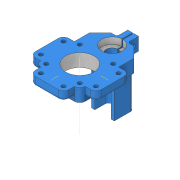
# Autodesk Inventor part: 1 gear box base
Saved by Autodesk Inventor 2020 (Build 240168000, 168)
## iProperties
Created: 2018-08-14
Part Number: 1 gear box base
Material: Generic
Document SubType Name: Modeling
Designer: mrbeh
Density: 1 g/cm^3
Appearance: Default
Author: mrbeh
Autodesk Inventor part; units mm, degrees
ref_plane "YZ Plane" through (0, 0, 0) normal (1, 0, 0) x (0, 1, 0)
ref_plane "XZ Plane" through (0, 0, 0) normal (0, 1, 0) x (-1, 0, 0)
ref_plane "XY Plane" through (0, 0, 0) normal (0, 0, 1) x (1, 0, 0)
sketch "Sketch1" plane through (0, 0, 0) normal (0, 1, 0) x (-1, 0, 0)
  line L0 (0, 0) -> (42, 0)
  line L1 (42, 0) -> (42, -60)
  line L2 (42, -60) -> (0, -60)
  line L3 (0, -60) -> (0, 0)
  dimension "d0" = 42
  dimension "d1" = 60
  constraints: 8 end point, 2 parallel, 1 horizontal, 1 perpendicular
  measures "d0" distance of L1.end L2.end
  measures "d1" distance of L0.end L1.end
extrude "Extrusion1" add sketch "Sketch1" along normal blind 12
sketch "Sketch2" plane through (0, 12, 0) normal (0, 1, 0) x (1, 0, 0)
  circle A0 centre (-5, 5) radius 1.8
  point P0 (0, 0)
  dimension "d4" = 3.6
  constraints: 1 centre point
  measures "d4" diameter of A0
extrude "Extrusion2" cut sketch "Sketch2" against normal blind 12
pattern_linear "Rectangular Pattern1" count 2 spacing 31 along (0, 0, -1) count 2 spacing 31 along (-1, 0, 0) of "Extrusion2"
sketch "Sketch3" plane through (0, 12, 0) normal (0, 1, 0) x (1, 0, 0)
  circle A0 centre (-20.5, 20.5) radius 11.5
  point P0 (0, 0)
  dimension "d13" = 23
  constraints: 1 centre point
  measures "d13" diameter of A0
extrude "Extrusion3" cut sketch "Sketch3" against normal blind 12
sketch "Sketch5" plane through (0, 0, 0) normal (0, -1, 0) x (1, 0, 0)
  line L0 (-42, -60) -> (0, -60) projected
  line L1 (0, -31.65) -> (-42, -31.65)
  line L2 (-42, -31.65) -> (-42, -60)
  line L3 (-42, -60) -> (0, -60)
  line L4 (0, -60) -> (0, -31.65)
  point P0 (0, 0)
  constraints: 8 end point, 2 parallel, 1 horizontal, 1 perpendicular
extrude "Extrusion5" add sketch "Sketch5" along normal blind 39.25
sketch "Sketch6" plane through (0, 12, 0) normal (0, 1, 0) x (1, 0, 0)
  line L0 (-25.5, 60) -> (-25.5, 70)
  line L1 (-25.5, 70) -> (-15.5, 70)
  line L2 (-15.5, 70) -> (-15.5, 60)
  line L3 (-42, 60) -> (0, 60) projected
  line L4 (-25.5, 60) -> (-15.5, 60)
  point P0 (0, 0)
  dimension "d21" = 10
  dimension "d23" = 10
  constraints: 8 end point, 2 point on line, 1 parallel
  measures "d21" distance of L0.end L1.end
  measures "d23" distance of L1.end L2.end
extrude "Extrusion6" add sketch "Sketch6" against normal blind 12
sketch "Sketch7" plane through (0, 12, 0) normal (0, 1, 0) x (1, 0, 0)
  line L0 (-20, 60.5) -> (-21, 60.5)
  line L1 (-21, 60.5) -> (-21, 81.6021)
  line L2 (-21, 81.6021) -> (-20, 81.6021)
  line L3 (-20, 81.6021) -> (-20, 60.5)
  point P0 (0, 0)
  dimension "d26" = 1
  constraints: 8 end point, 2 parallel, 1 horizontal, 1 perpendicular
  measures "d26" distance of L1.end L2.end
extrude "Extrusion7" cut sketch "Sketch7" against normal blind 12
sketch "Sketch10" plane through (-25.5, 12, -70) normal (-1, 0, 0) x (0, 0, 1)
  circle A0 centre (5, -6) radius 1.8
  point P0 (70, -12)
  dimension "d35" = 3.6
  constraints: 1 centre point
  measures "d35" diameter of A0
extrude "Extrusion10" cut sketch "Sketch10" against normal blind 10
sketch "Sketch12" plane through (0, 12, 0) normal (0, 1, 0) x (1, 0, 0)
  line L0 (-42, 60) -> (-42, 0) projected
  line L1 (-42, 60) -> (0, 60) projected
  line L2 (-42, 0) -> (-41, 0)
  line L3 (-41, 0) -> (-41, 60)
  line L4 (-41, 60) -> (-42, 60)
  line L5 (-42, 60) -> (-42, 0)
  point P0 (0, 0)
  dimension "d44" = 1
  constraints: 8 end point, 2 parallel, 1 horizontal, 1 perpendicular, 1 point on line
  measures "d44" distance of L4.end L3.end
extrude "Extrusion12" cut sketch "Sketch12" against normal blind 70
fillet "Fillet1" radius 2 2 edges at (-15.5, 6, -60) (-25.5, 6, -60)
fillet "Fillet3" radius 5 2 edges at (0, 6, 0) (-41, 6, 0)
chamfer "Chamfer1" distance 10 angle 45 2 edges at (0, -13.625, -60) (-41, -13.625, -60)
sketch "Sketch14" plane through (0, -39.25, -31.65) normal (0, 0, 1) x (1, 0, 0)
  line L0 (0, 39.25) -> (-5, 39.25) projected
  line L1 (0, 39.25) -> (-10, 39.25)
  line L2 (-10, 39.25) -> (-10, 3.175)
  line L3 (0, 3.175) -> (0, 39.25)
  line L4 (0, 39.25) -> (0, 0) projected
  line L5 (-10, 39.25) -> (0, 39.25)
  line L6 (0, 39.25) -> (0, 0)
  line L7 (0, 0) -> (-10, 0)
  line L8 (-10, 0) -> (-10, 39.25)
  dimension "d57" = 10
  constraints: 14 end point, 3 parallel, 2 horizontal, 2 perpendicular
  measures "d57" distance of L3.start L2.end
extrude "Extrusion14" cut sketch "Sketch14" against normal blind 30
ref_plane "Work Plane1" through (-20.5, 0, -5) normal (1, 0, 0) x (0, 0, -1)
mirror "Mirror1" about plane through (-20.5, 0, -5) normal (1, 0, 0) of "Extrusion14"
sketch "Sketch15" plane through (0, -39.25, 0) normal (0, -1, 0) x (1, 0, 0)
  line L0 (-31, -31.65) -> (-23.3156, -31.65) projected
  line L1 (-13, -31.65) -> (-28, -31.65)
  line L2 (-28, -31.65) -> (-28, -54.65)
  line L3 (-28, -54.65) -> (-13, -54.65)
  line L4 (-13, -54.65) -> (-13, -31.65)
  point P0 (0, 0)
  point P1 (-31, -41.65)
  point P2 (-10, -41.65)
  dimension "d61" = 15
  dimension "d62" = 23
  constraints: 8 end point, 2 parallel, 1 horizontal, 1 perpendicular, 2 other
  measures "d61" distance of L3.end L2.end
  measures "d62" distance of L2.end L1.end
extrude "Extrusion15" cut sketch "Sketch15" against normal blind 36
fillet "Fillet5" radius 3 4 edges at (-10, -19.625, -60) (-28, -21.25, -54.65) (-13, -21.25, -54.65) (-31, -19.625, -60)
sketch "Sketch16" plane through (0, 0, 0) normal (0, -1, 0) x (1, 0, 0)
  line L0 (-41, -50) -> (-41, -5) projected
  line L1 (0, 0) -> (-41, 0)
  line L2 (-41, 0) -> (-41, -42)
  line L3 (-41, -42) -> (0, -42)
  line L4 (0, -42) -> (0, 0)
  dimension "d66" = 42
  constraints: 8 end point, 2 parallel, 1 horizontal, 1 perpendicular, 1 point on line
  measures "d66" distance of L2.end L1.end
extrude "Extrusion16" cut sketch "Sketch16" along normal blind 50
sketch "Sketch17" plane through (0, 12, 0) normal (0, 1, 0) x (1, 0, 0)
  circle A0 centre (-20.5, 50.5) radius 8.55
  point P0 (0, 0)
  dimension "d69" = 17.1
  constraints: 1 centre point
  measures "d69" diameter of A0
extrude "Extrusion17" cut sketch "Sketch17" against normal blind 12.5
sketch "Sketch18" plane through (0, 12, 0) normal (0, 1, 0) x (1, 0, 0)
  line L0 (-25.5, 70) -> (-21, 70) projected
  line L1 (-21, 70) -> (-20, 70)
  line L2 (-20, 70) -> (-20, 46.0375)
  line L3 (-20, 46.0375) -> (-21, 46.0375)
  line L4 (-21, 46.0375) -> (-21, 70)
  point P0 (0, 0)
  constraints: 8 end point, 2 parallel, 1 horizontal, 1 perpendicular
extrude "Extrusion18" cut sketch "Sketch18" against normal blind 12.5
sketch "Sketch20" plane through (0, 12, 0) normal (0, 1, 0) x (1, 0, 0)
  line L0 (0, 50) -> (0, 5) projected
  line L1 (0, 36) -> (10, 36)
  line L2 (10, 36) -> (10, 5)
  line L3 (10, 5) -> (0, 5)
  line L4 (0, 5) -> (0, 36)
  point P0 (0, 0)
  dimension "d76" = 10
  constraints: 8 end point, 2 parallel, 1 horizontal, 1 perpendicular, 1 point on line
  measures "d76" distance of L2.end L3.end
extrude "Extrusion19" add sketch "Sketch20" against normal blind 8
pattern_circular "Circular Pattern2" count 3 over 180 about axis through (-20.5, 12, -20.5) along (0, -1, 0) of "Extrusion19"
sketch "Sketch21" plane through (0, 12, 0) normal (0, 1, 0) x (1, 0, 0)
  circle A0 centre (5, 31) radius 1.8
  point P0 (0, 0)
  dimension "d82" = 3.6
  constraints: 1 centre point
  measures "d82" diameter of A0
extrude "Extrusion20" cut sketch "Sketch21" against normal blind 8
pattern_linear "Rectangular Pattern2" count 2 spacing 21 along (0, 0, 1) of "Extrusion20"
pattern_circular "Circular Pattern3" count 3 over 180 about axis through (-20.5, 12, -20.5) along (0, -1, 0) of "Extrusion20", "Rectangular Pattern2"
fillet "Fillet6" radius 5 6 edges at (10, 8, -36) (10, 8, -5) (-5, 8, 10) (-36, 8, 10) (-51, 8, -5) (-51, 8, -36)
fillet "Fillet7" radius 2 5 edges at (-51, 4, -20.5) (-49.5355, 4, -34.5355) (-43.5, 4, -36) (-49.5355, 4, -6.4645) (-43.5, 4, -5)
fillet "Fillet8" radius 2 10 edges at (-20.5, 4, 10) (-34.5355, 4, 8.5355) (-36, 4, 2.5) (-6.4645, 4, 8.5355) (-5, 4, 2.5) (8.5355, 4, -6.4645) (2.5, 4, -5) (8.5355, 4, -34.5355) (2.5, 4, -36) (10, 4, -20.5)
sketch "Sketch22" plane through (0, 12, 0) normal (0, 1, 0) x (1, 0, 0)
  circle A0 centre (-20.5, 20.5) radius 11.5 projected
  circle A1 centre (-20.5, 20.5) radius 13
  point P0 (0, 0)
  dimension "d94" = 26
  constraints: 1 centre point, 1 coincident
  measures "d94" diameter of A1
extrude "Extrusion21" cut sketch "Sketch22" against normal blind 20
sketch "Sketch23" plane through (0, 4, 0) normal (0, -1, 0) x (1, 0, 0)
  circle A0 centre (5, -10) radius 1.8 projected
  line L0 (3.3834, -12.8) -> (1.7668, -10)
  line L1 (1.7668, -10) -> (3.3834, -7.2)
  line L2 (3.3834, -7.2) -> (6.6166, -7.2)
  line L3 (6.6166, -7.2) -> (8.2332, -10)
  line L4 (8.2332, -10) -> (6.6166, -12.8)
  line L5 (6.6166, -12.8) -> (3.3834, -12.8)
  point P0 (0, 0)
  point P1 (5, -12.8)
  constraints: 12 end point, 1 coincident, 1 midpoint, 13 other
extrude "Extrusion22" cut sketch "Sketch23" against normal blind 2.5
mirror "Mirror2" about plane through (-20.5, 0, -5) normal (1, 0, 0) of "Extrusion22"
ref_plane "Work Plane2" through (0, 12, -20.5) normal (0, 0, 1) x (1, 0, 0)
mirror "Mirror3" about plane through (0, 12, -20.5) normal (0, 0, 1) of "Extrusion22", "Mirror2"
sketch "Sketch24" plane through (-34, 4, 0) normal (0, -1, 0) x (1, 0, 0)
  circle A0 centre (24, 5) radius 1.8 projected
  line L0 (21.2, 6.6166) -> (24, 8.2332)
  line L1 (24, 8.2332) -> (26.8, 6.6166)
  line L2 (26.8, 6.6166) -> (26.8, 3.3834)
  line L3 (26.8, 3.3834) -> (24, 1.7668)
  line L4 (24, 1.7668) -> (21.2, 3.3834)
  line L5 (21.2, 3.3834) -> (21.2, 6.6166)
  point P0 (34, 0)
  point P1 (21.2, 5)
  constraints: 12 end point, 1 coincident, 1 midpoint, 13 other
extrude "Extrusion23" cut sketch "Sketch24" against normal blind 2.5
ref_plane "Work Plane3" through (-20.5, 12, 0) normal (-1, 0, 0) x (0, 0, 1)
mirror "Mirror4" about plane through (-20.5, 12, 0) normal (-1, 0, 0) of "Extrusion23"
sketch "Sketch25" plane through (0, 12, 0) normal (0, 1, 0) x (1, 0, 0)
  arc A0 (-21, 59.0354) -> (-20, 59.0354) centre (-20.5, 50.5) ccw projected
  circle A1 centre (-20.5, 50.5) radius 9.55
  point P0 (0, 0)
  dimension "d105" = 19.1
  constraints: 1 centre point, 1 coincident
  measures "d105" diameter of A1
extrude "Extrusion24" cut sketch "Sketch25" against normal blind 6
thicken "Thicken1" operation add thickness 3 both sides no extend neighbours yes toward (-0.2745218, 0, -0.9615809) faces at (-18.1528, 1.8333, -42.2785)
body "Solid1"
